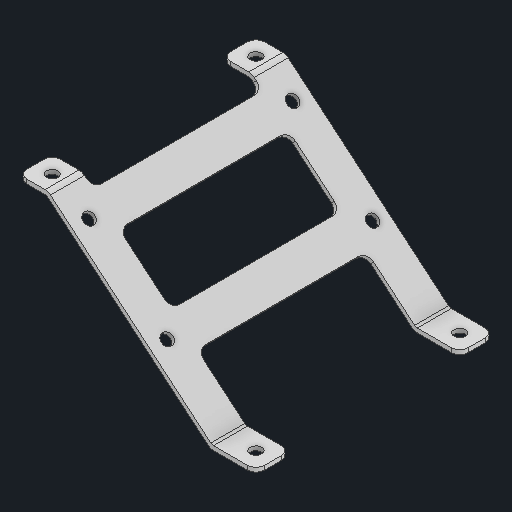
# Autodesk Inventor part: Brain Mount
Saved by Autodesk Inventor 2025 (Build 290162000, 162)
## iProperties
Created: 2025-02-04
Part Number: Brain Mount
Material: Generic
Document SubType Name: Modeling
Designer: Averey Ku
Density: 1 g/cm^3
Appearance: Default
Sheet Metal Rule: Default
Mass: 6.70374 g
Surface Area: 96.7104 cm^2
Volume: 6.70374 cm^3
Author: Averey Ku
Autodesk Inventor part; units mm, degrees
ref_plane "YZ Plane" through (0, 0, 0) normal (1, 0, 0) x (0, 1, 0)
ref_plane "XZ Plane" through (0, 0, 0) normal (0, 1, 0) x (-1, 0, 0)
ref_plane "XY Plane" through (0, 0, 0) normal (0, 0, 1) x (1, 0, 0)
sketch "Sketch1" plane through (0, 0, 0) normal (0, 1, 0) x (-1, 0, 0)
  circle A0 centre (0, 0) radius 2.1844
  circle A1 centre (0, -76.2) radius 2.1844
  line L0 (-6.35, 3.175) -> (-6.35, -3.175)
  line L1 (100.0162, -3.175) -> (100.0162, 3.175)
  line L2 (96.8412, 6.35) -> (-3.175, 6.35)
  arc A2 (-3.175, 6.35) -> (-6.35, 3.175) centre (-3.175, 3.175) ccw
  arc A3 (-6.35, -3.175) -> (-3.175, -6.35) centre (-3.175, -3.175) ccw
  line L3 (-3.175, -82.55) -> (96.8412, -82.55)
  line L4 (100.0162, -79.375) -> (100.0162, -73.025)
  line L5 (-6.35, -73.025) -> (-6.35, -79.375)
  arc A4 (-3.175, -69.85) -> (-6.35, -73.025) centre (-3.175, -73.025) ccw
  arc A5 (-6.35, -79.375) -> (-3.175, -82.55) centre (-3.175, -79.375) ccw
  line L6 (33.9344, -9.525) -> (33.9344, -66.675)
  line L7 (46.6344, -66.675) -> (46.6344, -9.525)
  line L8 (-3.175, -6.35) -> (30.7594, -6.35)
  line L9 (30.7594, -69.85) -> (-3.175, -69.85)
  circle A6 centre (40.2844, 0) radius 2.1844
  circle A7 centre (40.2844, -76.8593) radius 2.1844
  circle A8 centre (78.3844, 0) radius 2.1844
  circle A9 centre (78.378, -76.16) radius 2.1844
  circle A10 centre (93.6662, 0) radius 2.1844
  circle A11 centre (93.6662, -76.2) radius 2.1844
  arc A12 (100.0162, -73.025) -> (96.8412, -69.85) centre (96.8412, -73.025) ccw
  arc A13 (96.8412, -82.55) -> (100.0162, -79.375) centre (96.8412, -79.375) ccw
  arc A14 (96.8412, -6.35) -> (100.0162, -3.175) centre (96.8412, -3.175) ccw
  arc A15 (100.0162, 3.175) -> (96.8412, 6.35) centre (96.8412, 3.175) ccw
  line L10 (72.0344, -66.675) -> (72.0344, -9.525)
  line L11 (84.7344, -66.675) -> (84.7344, -9.525)
  line L12 (96.8412, -69.85) -> (87.9094, -69.85)
  line L13 (68.8594, -69.85) -> (49.8094, -69.85)
  line L14 (49.8094, -6.35) -> (68.8594, -6.35)
  line L15 (87.9094, -6.35) -> (96.8412, -6.35)
  arc A16 (84.7344, -66.675) -> (87.9094, -69.85) centre (87.9094, -66.675) ccw
  arc A17 (68.8594, -69.85) -> (72.0344, -66.675) centre (68.8594, -66.675) ccw
  arc A18 (72.0344, -9.525) -> (68.8594, -6.35) centre (68.8594, -9.525) ccw
  arc A19 (87.9094, -6.35) -> (84.7344, -9.525) centre (87.9094, -9.525) ccw
  arc A20 (49.8094, -6.35) -> (46.6344, -9.525) centre (49.8094, -9.525) ccw
  arc A21 (46.6344, -66.675) -> (49.8094, -69.85) centre (49.8094, -66.675) ccw
  arc A22 (30.7594, -69.85) -> (33.9344, -66.675) centre (30.7594, -66.675) ccw
  arc A23 (33.9344, -9.525) -> (30.7594, -6.35) centre (30.7594, -9.525) ccw
  point P0 (-6.35, -6.35)
  point P1 (100.0162, -6.35)
  point P2 (100.0162, 6.35)
  point P3 (100.0162, -82.55)
  point P4 (100.0162, -69.85)
  point P5 (33.9344, -6.35)
  point P6 (33.9344, -69.85)
  point P7 (46.6344, -69.85)
  point P8 (46.6344, -6.35)
  point P9 (100.0162, -76.2)
  dimension "d0" = 4.3688
  dimension "d1" = 4.3688
  dimension "d3" = 3.175
  dimension "d4" = 3.175
  dimension "d15" = 4.3688
  dimension "d16" = 106.3662
  dimension "d17" = 3.175
  dimension "d18" = 6.35
  dimension "d19" = 12.7
  dimension "d23" = 106.3662
  dimension "d24" = 3.175
  dimension "d25" = 38.1
  dimension "d27" = 38.1
  dimension "d28" = 12.7
  dimension "d29" = 6.35
  constraints: 38 tangent, 32 end point, 32 point on circle, 24 centre point, 21 perpendicular, 15 point on line, 12 equal radius, 3 vertical, 1 coincident, 1 horizontal, 1 midpoint
  measures "d0" diameter of A0
  measures "d1" diameter of A1
  measures "d3" radius of A2
  measures "d4" radius of A4
  measures "d15" diameter of A10
  measures "d16" distance between parallel lines of L4 L5
  measures "d17" radius of A12
  measures "d18" distance from line of L7 A6.centre
  measures "d19" distance between parallel lines of L7 L6
  measures "d23" distance between parallel lines of L0 L1
  measures "d24" radius of A16
  measures "d25" distance of A6.centre A8.centre
  measures "d27" distance of A7.centre A9.centre
  measures "d28" distance between parallel lines of L10 L11
  measures "d29" distance from line of L11 A8.centre
extrude "Extrusion1" add sketch "Sketch1" along normal blind 1.5875
sketch "Sketch2" plane through (0, 1.5875, 0) normal (0, 1, 0) x (1, 0, 0)
  line L0 (-9.525, -6.35) -> (-9.525, 82.55)
  line L1 (3.175, 82.55) -> (-96.8412, 82.55) projected
  point P0 (0, 0)
  point P1 (-95.3556, 82.55)
  dimension "d7" = 9.525
  constraints: 2 end point, 1 point on line, 1 vertical
  measures "d7" distance from line of point (0, 0) L0
bend part "Bend Part2" radius 1.5875 angle 40 line through (-9.525, 1.5875, 6.35) along (0, 0, -1) centre toward (0, 1, 0) moving side (-1, 0, 0) both sides no
sketch "Sketch4" plane through (-39.1443, 23.8839, -69.85) normal (-0.6427876, -0.7660444, 0) x (0.7660444, -0.6427876, 0)
  line L0 (36.0011, -12.7) -> (-50.2068, -12.7) projected
  line L1 (-42.2656, -12.7) -> (-42.2656, 76.2)
  line L2 (-53.3818, 66.675) -> (-53.3818, 73.025) projected
  point P0 (45.3385, 69.85)
  point P1 (-57.2556, -12.7)
  point P2 (-53.3818, 69.85)
  dimension "d26" = 11.1162
  constraints: 2 end point, 1 midpoint, 1 point on line, 1 vertical
  measures "d26" distance from line of L1 point (-53.382, 69.85)
bend part "Bend Part3" radius 1.5875 angle 40 line through (-71.5216, 51.0517, -82.55) along (0, 0, 1) centre toward (-0.6427876, -0.7660444, 0) moving side (-0.7660444, 0.6427876, 0) both sides no
equation "\"BendRadius\" = Thickness"
equation "\"BendReliefWidth\" = Thickness"
equation "\"BendReliefDepth\" = 0.5 * Thickness"
equation "\"CornerReliefSize\" = 4 * Thickness"
equation "\"MinimumRemnant\" = 2 * Thickness"
equation "\"TransitionRadius\" = BendRadius"
equation "\"JacobiRadiusSize\" = BendRadius"
equation "\"GapSize\" = Thickness"
equation "\"Thickness\" = 3.048"
body "Solid1"
